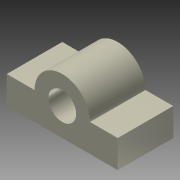
# Autodesk Inventor part: proxybearing
Saved by Autodesk Inventor 2011 SP1 (Build 150282100, 282)
## iProperties
Created: 2012-01-20
Part Number: proxybearing
Document SubType Name: Modeling
Designer: Christopher
Density: 1 g/cm^3
Author: Christopher
Autodesk Inventor part; units mm, degrees
ref_plane "YZ Plane" through (0, 0, 0) normal (1, 0, 0) x (0, 1, 0)
ref_plane "XZ Plane" through (0, 0, 0) normal (0, 1, 0) x (-1, 0, 0)
ref_plane "XY Plane" through (0, 0, 0) normal (0, 0, 1) x (1, 0, 0)
sketch "Sketch1" plane through (0, 0, 0) normal (0, 0, 1) x (1, 0, 0)
  line L0 (-19.4444, 0) -> (31.3556, 0)
  line L1 (31.3556, 0) -> (31.3556, 12.7)
  line L2 (31.3556, 12.7) -> (-19.4444, 12.7)
  line L3 (-19.4444, 12.7) -> (-19.4444, 0)
  circle A0 centre (5.9556, 12.7) radius 6.35
  circle A1 centre (5.9556, 12.7) radius 12.7
  point P0 (0, 0)
  dimension "d0" = 50.8
  dimension "d2" = 12.7
  dimension "d3" = 12.7
  dimension "d4" = 25.4
  constraints: 8 end point, 2 centre point, 2 parallel, 1 coincident, 1 horizontal, 1 perpendicular
  measures "d0" distance of L0.start L0.end
  measures "d2" distance between parallel lines of L0 L2
  measures "d3" diameter of A0
  measures "d4" diameter of A1
extrude "Extrusion1" add sketch "Sketch1" against normal blind 25.4 contours L3 L2 A1 L0 | A1 L2 L1 L0 | A1 L2 A0 | A1 L2 A0 | L2 A0 picked at (5.205, 10.7209)
extrude "Extrusion2" cut sketch "Sketch1" against normal blind 25.4 contours A0 L2 | L2 A0
body "Solid1"
